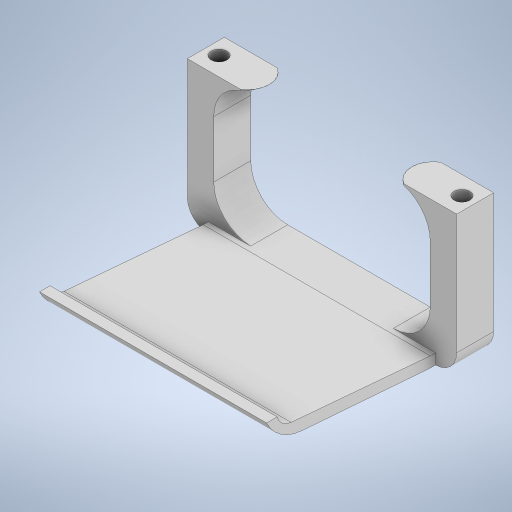
# Autodesk Inventor part: SAW_clamp_sled
Saved by Autodesk Inventor 2024.2 (Build 282272000, 272)
## iProperties
Created: 2024-05-24
Part Number: SAW_clamp_sled
Material: Generic
Document SubType Name: Modeling
Designer: magn1
Density: 1 g/cm^3
Appearance: Default
Author: magn1
Autodesk Inventor part; units mm, degrees
ref_plane "YZ Plane" through (0, 0, 0) normal (1, 0, 0) x (0, 1, 0)
ref_plane "XZ Plane" through (0, 0, 0) normal (0, 1, 0) x (-1, 0, 0)
ref_plane "XY Plane" through (0, 0, 0) normal (0, 0, 1) x (1, 0, 0)
sketch "Sketch1" plane through (0, 0, 0) normal (0, 0, 1) x (1, 0, 0)
  line L0 (-20.5, -12.375) -> (20.5, -12.375)
  line L1 (20.5, -12.375) -> (20.5, 12.375)
  line L2 (20.5, 12.375) -> (-20.5, 12.375)
  line L3 (-20.5, 12.375) -> (-20.5, -12.375)
  line L4 (-20.5, -12.375) -> (20.5, 12.375) construction
  line L5 (20.5, -12.375) -> (-20.5, 12.375) construction
  line L6 (-20.5, 12.375) -> (-25.5, 12.375) construction
  line L7 (20.5, 12.375) -> (25.5, 12.375) construction
  line L8 (20.5, -12.375) -> (25.5, -12.375) construction
  line L9 (25.5, -12.375) -> (25.5, -14.375) construction
  line L10 (-25.5, 12.375) -> (25.5, 12.375)
  line L11 (25.5, 12.375) -> (25.5, -14.375)
  line L12 (25.5, -14.375) -> (-25.5, -14.375)
  line L13 (-25.5, -14.375) -> (-25.5, 12.375)
  line L14 (-20.5, 12.375) -> (-13.5, 12.375)
  line L15 (20.5, 12.375) -> (13.5, 12.375)
  line L16 (13.5, 12.375) -> (13.5, 5.375) construction
  line L17 (-13.5, 12.375) -> (-13.5, 5.375) construction
  circle A0 centre (-13.5, 5.375) radius 7
  circle A1 centre (13.5, 5.375) radius 7
  point P0 (0, 0)
  point P1 (-20.5, 5.375)
  point P2 (20.5, 12.375)
  point P3 (20.5, 5.375)
  dimension "d0" = 41
  dimension "d3" = 24.75
  dimension "d4" = 5
  dimension "d5" = 5
  dimension "d6" = 5
  dimension "d7" = 2
  dimension "d8" = 7
  dimension "d9" = 7
  dimension "d10" = 7
  dimension "d11" = 7
  constraints: 36 end point, 5 horizontal, 5 perpendicular, 4 parallel, 2 coincident, 2 midpoint, 2 point on line, 6 other
  measures "d0" distance of L2.end L1.end
  measures "d3" distance between parallel lines of L0 L2
  measures "d4" distance of L2.end L6.end
  measures "d5" distance of L1.end L7.end
  measures "d6" distance of L0.end L8.end
  measures "d7" distance of L8.end L9.end
  measures "d8" distance of L2.end L14.end
  measures "d9" distance of L1.end L15.end
  measures "d10" distance of L15.end L16.end
  measures "d11" distance of L14.end L17.end
extrude "Extrusion1" add sketch "Sketch1" along normal blind 7 contours L0 L1 L10 L11 L12 L13 L3 | L3 L2 A0 | A1 L2 L1
fillet "Fillet1" radius 7 2 edges at (-20.5, -12.375, 3.5) (20.5, -12.375, 3.5)
fillet "Fillet2" radius 4 2 edges at (-25.5, -14.375, 3.5) (25.5, -14.375, 3.5)
sketch "Sketch2" plane through (-25.5, 12.375, 0) normal (0, 1, 0) x (1, 0, 0)
  line L0 (0, 0) -> (2.5, 0) construction
  line L1 (12, 0) -> (0, 0) construction
  line L2 (2.5, 0) -> (2.5, -3.5) construction
  line L3 (12, -7) -> (0, -7) construction
  circle A0 centre (2.5, -3.5) radius 1.5
  line L4 (51, 0) -> (51, -7) construction
  line L5 (51, 0) -> (48.5, 0) construction
  line L6 (51, 0) -> (39, 0) construction
  line L7 (48.5, 0) -> (48.5, -3.5) construction
  circle A1 centre (48.5, -3.5) radius 1.5
  point P0 (25.5, 0)
  dimension "d16" = 2.5
  dimension "d17" = 3.5
  dimension "d18" = 3
  dimension "d19" = 2.5
  dimension "d20" = 3.5
  dimension "d21" = 3
  constraints: 8 end point, 2 centre point, 2 coincident, 2 perpendicular, 2 point on line
  measures "d16" distance of L0.start L0.end
  measures "d17" distance of L0.end L2.end
  measures "d18" diameter of A0
  measures "d19" distance of L4.start L5.end
  measures "d20" distance of L5.end L7.end
  measures "d21" diameter of A1
extrude "Extrusion2" cut sketch "Sketch2" against normal blind 7
sketch "Sketch3" plane through (0, 0, 7) normal (0, 0, 1) x (1, 0, 0)
  arc A0 (-20.5, -5.375) -> (-13.5, -12.375) centre (-13.5, -5.375) ccw projected
  arc A1 (-25.5, -10.375) -> (-21.5, -14.375) centre (-21.5, -10.375) ccw projected
  line L0 (-13.5, -12.375) -> (-21.5, -12.375)
  line L1 (-21.5, -12.375) -> (-21.5, -14.375)
  line L2 (-21.5, -14.375) -> (-13.5, -14.375)
  line L3 (-13.5, -14.375) -> (-13.5, -12.375)
  line L4 (13.5, -12.375) -> (-13.5, -12.375) projected
  line L5 (-21.5, -14.375) -> (21.5, -14.375) projected
  line L6 (13.5, -12.375) -> (21.5, -12.375)
  line L7 (21.5, -12.375) -> (21.5, -14.375)
  line L8 (21.5, -14.375) -> (13.5, -14.375)
  line L9 (13.5, -14.375) -> (13.5, -12.375)
  line L10 (-13.5, -12.375) -> (13.5, -12.375)
  line L11 (13.5, -12.375) -> (13.5, -14.375)
  line L12 (13.5, -14.375) -> (-13.5, -14.375)
  line L13 (-13.5, -14.375) -> (-13.5, -12.375)
  point P0 (0, 0)
  dimension "d24" = 8
  constraints: 24 end point, 6 parallel, 3 horizontal, 3 perpendicular
  measures "d24" distance of L5.end L8.end
extrude "Extrusion3" add sketch "Sketch3" along normal blind 1
sketch "Sketch7" plane through (-21.5, -14.375, 7) normal (-1, 0, 0) x (0, 0, 1)
  line L0 (1, 0) -> (30, 0) construction
  line L1 (30, 0) -> (30, 4.5) construction
  line L2 (1, 2) -> (30, 4.5)
  line L3 (1, 0) -> (30, 2.25)
  line L4 (30, 4.5) -> (30, 6.5)
  line L5 (30, 6.5) -> (32, 6.5)
  line L6 (32, 6.5) -> (32, 2.4052)
  line L7 (32, 2.4052) -> (30, 2.25)
  line L8 (1, 0) -> (1, 2)
  point P0 (-7, 14.375)
  dimension "d42" = 29
  dimension "d43" = 4.5
  dimension "d44" = 2
  dimension "d45" = 2
  constraints: 18 end point, 3 vertical, 2 perpendicular, 1 collinear, 1 horizontal, 1 midpoint
  measures "d42" distance of L0.start L0.end
  measures "d43" distance of L0.end L1.end
  measures "d44" distance of L1.end L4.end
  measures "d45" distance of L4.end L5.end
extrude "Extrusion6" add sketch "Sketch7" against normal up to surface (43 mm away)
fillet "Fillet3" radius 8 1 edges at (0, -11.9698, 39)
fillet "Fillet4" radius 3 1 edges at (0, -9.875, 37)
sketch "Sketch8" plane through (-25.5, 12.375, 0) normal (0, 1, 0) x (1, 0, 0)
  line L0 (0, 0) -> (0, -7) projected
  line L1 (39, 0) -> (12, 0) projected
  line L2 (0, -7) -> (12, -7)
  line L3 (12, -7) -> (12, 0)
  line L4 (12, 0) -> (0, 0)
  line L5 (0, 0) -> (0, -7)
  line L6 (39, 0) -> (39, -7) projected
  line L7 (51, 0) -> (51, -7) projected
  line L8 (39, 0) -> (51, 0)
  line L9 (51, 0) -> (51, -7)
  line L10 (51, -7) -> (39, -7)
  line L11 (39, -7) -> (39, 0)
  circle A0 centre (48.5, -3.5) radius 1.5 projected
  circle A1 centre (48.5, -3.5) radius 1.5
  circle A2 centre (2.5, -3.5) radius 1.5 projected
  circle A3 centre (2.5, -3.5) radius 1.5
  line L12 (12, -7) -> (10, -7) construction
  line L13 (10, -7) -> (10, 0) construction
  line L14 (39, -7) -> (41, -7) construction
  line L15 (41, -7) -> (41, 0) construction
  arc A4 (10, -7) -> (10, 0) centre (7.9375, -3.5) ccw
  arc A5 (41, 0) -> (41, -7) centre (43.0625, -3.5) ccw
  point P0 (25.5, 0)
  point P1 (39, -3.5)
  point P2 (12, -3.5)
  dimension "d52" = 2
  dimension "d53" = 2
  dimension "d54" = 3
  dimension "d55" = 3
  constraints: 24 end point, 4 centre point, 4 parallel, 4 perpendicular, 4 point on circle, 4 point on line, 2 coincident, 2 horizontal, 2 tangent
  measures "d52" distance of L2.end L12.end
  measures "d53" distance of L10.end L14.end
  measures "d54" diameter of A1
  measures "d55" diameter of A3
extrude "Extrusion7" cut sketch "Sketch8" against normal blind 1 contours L4 L3 A4 | A4 L3 L2 | L8 A5 L6 | A5 L10 L6
body "Solid1"
